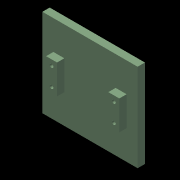
# Autodesk Inventor part: Table
Saved by Autodesk Inventor 2020 (Build 240168000, 168)
## iProperties
Created: 2019-08-12
Part Number: Table
Document SubType Name: Modeling
Designer: Administrator
Density: 1 g/cm^3
Mass: 1.31696 g
Surface Area: 15.9808 cm^2
Volume: 1.31696 cm^3
Material: 一般
Appearance: Green Pastel
Author: Administrator
Autodesk Inventor part; units mm, degrees
ref_plane "YZ Plane" through (0, 0, 0) normal (1, 0, 0) x (0, 1, 0)
ref_plane "XZ Plane" through (0, 0, 0) normal (0, 1, 0) x (-1, 0, 0)
ref_plane "XY Plane" through (0, 0, 0) normal (0, 0, 1) x (1, 0, 0)
sketch "Sketch1" plane through (0, 0, 0) normal (0, 0, 1) x (1, 0, 0)
  line L0 (0, 0) -> (10, 0) construction
  line L1 (0, 0) -> (0, 21.2479) construction
  line L2 (10, 0) -> (7, 0)
  line L3 (7, 0) -> (7, 2)
  line L4 (7, 2) -> (0, 2)
  line L5 (10, 0) -> (10, 2)
  line L6 (10, 2) -> (13, 2)
  line L7 (13, 2) -> (13, 4)
  line L8 (13, 4) -> (0, 4)
  line L9 (-7, 0) -> (-7, 2)
  line L10 (-7, 2) -> (0, 2)
  line L11 (-10, 0) -> (-10, 2)
  line L12 (-10, 2) -> (-13, 2)
  line L13 (-13, 2) -> (-13, 4)
  line L14 (-13, 4) -> (0, 4)
  line L15 (-10, 0) -> (-7, 0)
  line L16 (7, 0) -> (10, 0)
  dimension "d0" = 10
  dimension "d1" = 3
  dimension "d2" = 2
  dimension "d3" = 2
  dimension "d4" = 3
  dimension "d5" = 2
  constraints: 34 end point, 6 perpendicular, 6 symmetric about line, 3 point on line, 2 parallel, 1 collinear, 1 horizontal, 1 other
  measures "d0" distance of L0.start L0.end
  measures "d1" distance between parallel lines of L3 L5
  measures "d2" distance between parallel lines of L8 L6
  measures "d3" distance between parallel lines of L8 L4
  measures "d4" distance of L5.end L6.end
  measures "d5" distance between parallel lines of L4 L0
extrude "Extrusion1" add sketch "Sketch1" along normal mid plane 8
sketch "Sketch2" plane through (-10, 0, 4) normal (0, -1, 0) x (1, 0, 0)
  line L0 (3, -8) -> (3, 0) projected
  line L1 (17, -8.5525) -> (20, -8.5525) construction
  line L2 (20, 0.5525) -> (17, 0.5525) construction
  line L3 (0, 0) -> (0, -8) construction
  line L4 (0, -8) -> (3, -8) construction
  line L5 (3, -8) -> (3, 0) construction
  line L6 (3, 0) -> (0, 0) construction
  line L7 (1.5, 0) -> (1.5, -8) construction
  line L8 (18.5, 0.5525) -> (18.5, -8.5525) construction
  line L9 (1.5, -4) -> (18.5, -4) construction
  circle A0 centre (1.5, -1.5) radius 0.5
  line L10 (10, -4) -> (10, 0.5233) construction
  line L11 (18.5, -8.5525) -> (18.5, 0.5525) construction
  circle A1 centre (1.5, -6.5) radius 0.5
  circle A2 centre (18.5, -1.5) radius 0.5
  circle A3 centre (18.5, -6.5) radius 0.5
  line L12 (20, 0) -> (17, 0) projected
  line L13 (17, -8) -> (17, 0) projected
  line L14 (17, -8) -> (20, -8) projected
  line L15 (20, 0) -> (20, -8) projected
  line L16 (3, -4) -> (17, -4) construction
  line L17 (10, -4) -> (10, -13.0103) construction
  dimension "d8" = 1
  dimension "d9" = 2.5
  dimension "d10" = 0
  dimension "d11" = 0
  dimension "d12" = 8.5
  constraints: 26 end point, 10 midpoint, 5 symmetric about line, 4 centre point, 2 perpendicular, 1 point on line, 3 other
  measures "d8" diameter of A0
  measures "d9" distance from line of A0.centre L9
  measures "d10" distance between parallel lines of L17 L10
  measures "d11" distance between parallel lines of L16 L9
  measures "d12" distance between parallel lines of L10 L7
extrude "Extrusion2" cut sketch "Sketch2" against normal through all contours A0 | A1 | A2 | A3
sketch "Sketch3" plane through (-13, 4, 4) normal (0, 1, 0) x (1, 0, 0)
  circle A0 centre (21.5, 6.5) radius 0.5 projected
  circle A1 centre (21.5, 1.5) radius 0.5 projected
  circle A2 centre (4.5, 6.5) radius 0.5 projected
  circle A3 centre (4.5, 1.5) radius 0.5 projected
  circle A4 centre (4.5, 6.5) radius 1.1
  circle A5 centre (4.5, 1.5) radius 1.1
  circle A6 centre (21.5, 6.5) radius 1.1
  circle A7 centre (21.5, 1.5) radius 1.1
  dimension "d15" = 2.2
  constraints: 4 centre point, 3 equal radius
  measures "d15" diameter of A6
extrude "Extrusion3" cut sketch "Sketch3" against normal blind 1.2
sketch "Sketch4" plane through (-13, 4, 4) normal (0, 1, 0) x (1, 0, 0)
  line L0 (0, 8) -> (0, 0) projected
  line L1 (0, 8) -> (26, 8)
  line L2 (26, 8) -> (26, 16)
  line L3 (26, 16) -> (0, 16)
  line L4 (0, 16) -> (0, 8)
  line L5 (0, 0) -> (26, 0)
  line L6 (26, 0) -> (26, -8)
  line L7 (26, -8) -> (0, -8)
  line L8 (0, -8) -> (0, 0)
  constraints: 16 end point, 4 parallel, 2 collinear, 2 horizontal, 2 perpendicular
extrude "Extrusion4" add sketch "Sketch4" against normal up to surface (2 mm away)
